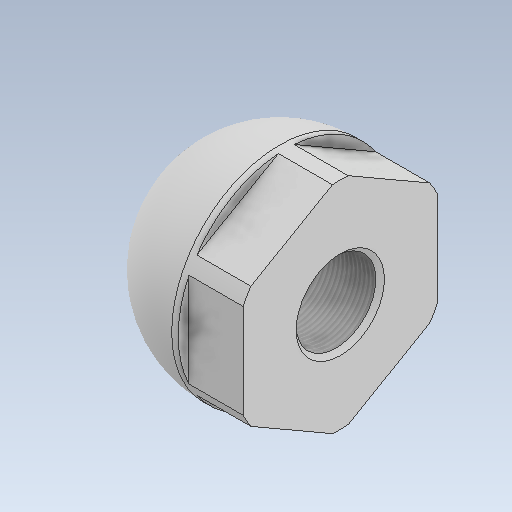
# Autodesk Inventor part: Peça37
Saved by Autodesk Inventor 2021 (Build 250183000, 183)
## iProperties
Category: 41
Created: 2021-07-21
Part Number: Peça37
Material: Genérico
Document SubType Name: Modeling
Designer: Giovanni
Density: 1 g/cm^3
Appearance: Padrão
User Status: 1:2
Author: Giovanni
Keywords: 37
Autodesk Inventor part; units mm, degrees
ref_plane "YZ Plane" through (0, 0, 0) normal (1, 0, 0) x (0, 1, 0)
ref_plane "XZ Plane" through (0, 0, 0) normal (0, 1, 0) x (-1, 0, 0)
ref_plane "XY Plane" through (0, 0, 0) normal (0, 0, 1) x (1, 0, 0)
sketch "Esboço1" plane through (0, 0, 0) normal (0, 0, 1) x (1, 0, 0)
  line L0 (0, 0) -> (-78, 0)
  arc A0 (-28, 50) -> (-78, 0) centre (-28, 0) ccw
  line L1 (-28, 50) -> (0, 50)
  line L2 (0, 50) -> (0, 0)
  line L3 (-106.0264, 0) -> (17.6711, 0) projected
  dimension "d0" = 28
  dimension "d1" = 50
  dimension "d2" = 50
  constraints: 6 end point, 2 horizontal, 2 point on circle, 1 centre point, 1 perpendicular, 1 point on line
  measures "d0" distance of L0.start A0.centre
  measures "d1" radius of A0
  measures "d2" distance of L0.start L1.end
revolve "Revolução1" add sketch "Esboço1" angle 360 about axis through (-10, 0, 0) along (1, 0, 0)
sketch "Esboço2" plane through (0, 0, 0) normal (1, 0, 0) x (0, 0, -1)
  point P0 (0, 0)
  point P1 (0, 0)
  constraints: 1 coincident
hole "Furo1" at (0, 0, 0) direction (-1, 0, 0) diameter 36.835 depth 50 tip angle 118 thread size "M39x2" class "6H" standard "ANSI Metric M Profile"
chamfer "Chanfro1" distance 2 angle 45 1 edges at (0, 0, 18.4175)
sketch "Esboço3" plane through (0, 0, 0) normal (1, 0, 0) x (0, 0, -1)
  circle A0 centre (0, 0) radius 50 projected
  circle A1 centre (0, 0) radius 20.4175 projected
  line L0 (45, 21.7945) -> (45, -21.7945)
  arc A2 (45, -21.7945) -> (45, 21.7945) centre (0, 0) ccw
  dimension "d14" = 45
  constraints: 4 point on circle, 2 end point, 1 centre point, 1 coincident, 1 concentric, 1 vertical
  measures "d14" distance from line of L0 A0.centre
extrude "Extrusão1" cut sketch "Esboço3" against normal blind 25 contours A0 L0 picked at (45.9189, -4.9362)
pattern_circular "Padrão circular1" count 6 over 360 about axis through (-10, 0, 0) along (1, 0, 0) of "Extrusão1"
